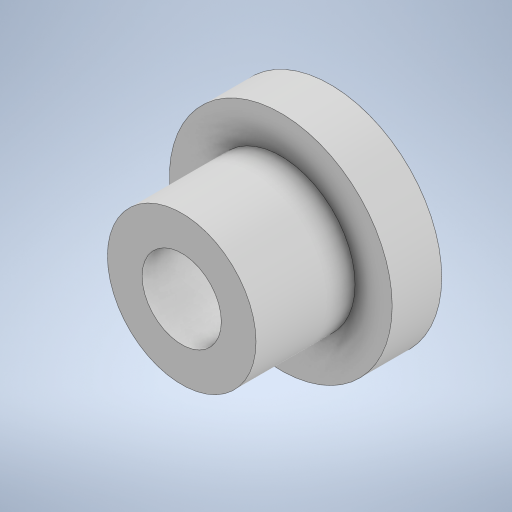
# Autodesk Inventor part: base-bearing-cap
Saved by Autodesk Inventor 2024 (Build 280153000, 153)
## iProperties
Created: 2024-02-09
Part Number: base-bearing-cap
Material: Generic
Document SubType Name: Modeling
Designer: MaartenGeorgesBuelen
Density: 1 g/cm^3
Appearance: Default
Author: MaartenGeorgesBuelen
## iProperties of the stored document base-bearing-cap_3DPrint.ipt
Created: 2024-02-22
Part Number: base-bearing-cap_3DPrint
Material: Generic
Document SubType Name: Modeling
Designer: MaartenGeorgesBuelen
Density: 1 g/cm^3
Appearance: Default
Author: MaartenGeorgesBuelen
Autodesk Inventor part; units mm, degrees
ref_plane "YZ Plane" through (0, 0, 0) normal (1, 0, 0) x (0, 1, 0)
ref_plane "Work Plane1" through (0, 0, -24) normal (0, 0, 1) x (1, 0, 0)
sketch "Sketch1" plane through (0, 0, -24) normal (0, 0, 1) x (1, 0, 0)
  circle A0 centre (0, 0) radius 6 projected
  circle A1 centre (0, 0) radius 9
  circle A2 centre (0, 0) radius 2.8
  point P0 (0, 0)
  dimension "d0" = 18
  dimension "d1" = 5.6
  constraints: 2 centre point, 2 coincident
  measures "d0" diameter of A1
  measures "d1" diameter of A2
extrude "Extrusion1" add sketch "Sketch1" along normal blind 4 contours A0 | A1
sketch "Sketch2" plane through (0, 0, -24) normal (0, 0, -1) x (-1, 0, 0)
  circle A0 centre (0, 0) radius 6
  circle A1 centre (0, 0) radius 2.8 projected
  circle A2 centre (0, 0) radius 3.2
  point P0 (0, 0)
  dimension "d4" = 12
  dimension "d5" = 0.4
  constraints: 2 centre point, 1 coincident
  measures "d4" diameter of A0
  measures "d5" radial gap between concentric circles of A1 A2
ref_plane "Work Plane2" through (-9.4625, -9.4625, -12) normal (0, 0, 1) x (0.9986, -0.0528, 0)
extrude "Extrusion2" add sketch "Sketch2" against normal up to surface (12 mm away) contours A0
body "Solid1"
